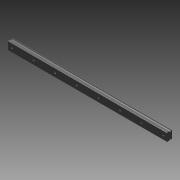
# Autodesk Inventor part: LU15AL294K2720100_rail
Saved by Autodesk Inventor 2011 SP1 (Build 150282100, 282)
## iProperties
Created: 2015-07-20
Part Number: LU15AL294K2720100_rail
Catalog Web Link: www.cadenas.de
Description: lu_rail-lu_rail
Vendor: NSK_RB
Document SubType Name: Modeling
Designer: PARTuser1
Manufacturer: NSK_RB
Mass: 37.8493 g
Surface Area: 162.952 cm^2
Volume: 37.8493 cm^3
Density: 1 g/cm^3
Category: PARTsolutions
Company: NSK_RB
Title: LU15AL
Author: Cadenas PARTsolutions
Comments: lu_rail
PSOL_IDENT_0: {$CADENAS_DATA\23d-libs\nsk_rb\nsk_linear_products\nsk_linear_guides\standard_series\lu_series\lu_al
PSOL_IDENT_1: _series\parts\lu_rail.prj},194 {VTYP=3D},{NB=LU15AL294K2720100_rail},{LINA=LU15AL},{NN=lu_rail},{DAT
PSOL_IDENT_2: E=17.04.2014 07:53:46},{GEOMDATE=17.04.2014 07:53:00},{VERSION=},{LINEID=740},{LINESUBID=-1},{WBVAR=
PSOL_IDENT_3: MAT,NOS,L0,G,POS1,POS2}  {NB=LU15AL294K2720100_rail},{LINA=LU15AL},{KT=DUMMY},{PN=LU15AL294K2720100_
PSOL_IDENT_4: rail},{MN=LU15AL},{ALG=LU15AL},{MNA=AL},{S=15},{MAT=K},{NOS=2},{L0=294},{G=7},{POS1=20},{POS2=100},{
PSOL_IDENT_5: MAT1='C','Special High carbon steel', 'K','Stainless steel'},{H=16.0},{E=4.0},{W2=8.5},{W=32},{L=43.
PSOL_IDENT_6: 600},{B=25},{J=20},{M=3.0},{TL=4.0},{B1=3.5},{L1=27.000},{J1=3.40},{K=12.0},{W1=15},{H1=9.5},{F=40},
PSOL_IDENT_7: {D=3.500},{DD=6.000},{HH=4.500},{B3=7.5},{G1=15.0},{GALGMIN=4},{GALGMAX=26.666667},{LMAX=1000},{LMIN=
PSOL_IDENT_8: 107.2},{NOMH=7},{POS1MIN=0},{POS1MAX=206.8},{POS2MIN=63.6},{POS2MAX=250.4},{DT=3.5},{DDT=6},{HHT=4.5
PSOL_IDENT_9: }
SUPPLIER: NSK_RB
ARTICLENO: LU15AL294K2720100_rail
BOMINFO: LU15AL
CREATOR: CADENAS GmbH
Autodesk Inventor part; units mm, degrees
sketch "Sketch_11" plane through (0, 0, 0) normal (1, 0, 0) x (0, 1, 0)
  line L0 (5, 7.5) -> (4.1225, 7.5)
  arc A0 (0.9321, 7.25) -> (4.1225, 7.5) centre (2.5175, 7.5) ccw
  line L1 (0.9321, 7.25) -> (0.25, 7.25)
  line L2 (0.25, 7.25) -> (0, 7.5)
  line L3 (0, 7.5) -> (-3.5, 7.5)
  line L4 (-3.5, 7.5) -> (-4, 7)
  line L5 (-4, 7) -> (-4, -6.9999)
  line L6 (-4, -6.9999) -> (-3.5, -7.5)
  line L7 (-3.5, -7.5) -> (0, -7.5)
  line L8 (0, -7.5) -> (0.25, -7.25)
  line L9 (0.25, -7.25) -> (0.9321, -7.25)
  arc A1 (4.1225, -7.5) -> (0.9321, -7.25) centre (2.5175, -7.5) ccw
  line L10 (4.1225, -7.5) -> (5, -7.5)
  line L11 (5, -7.5) -> (5.5, -7)
  line L12 (5.5, -7) -> (5.5, 7)
  line L13 (5.5, 7) -> (5, 7.5)
  constraints: 28 end point, 4 point on circle, 2 centre point
extrude "Extrusion1" add sketch "Sketch_11" along normal blind 294
sketch "Sketch_17" plane through (0, 0, 0) normal (0, 0, 1) x (1, 0, 0)
  line L0 (7, -4.5) -> (7, 6)
  line L1 (7, 6) -> (10, 6)
  line L2 (10, 6) -> (10, 1)
  line L3 (10, 1) -> (8.75, 1)
  line L4 (8.75, 1) -> (8.75, -4.5)
  line L5 (8.75, -4.5) -> (7, -4.5)
  line L6 (7, -4.5) -> (7, 6)
  constraints: 14 end point
revolve "Revolution1" cut sketch "Sketch_17" angle 360 about axis through (7, -4.5, 0) along (0, -1, 0)
pattern_linear "Rectangular Pattern1" count 8 spacing 40 along (1, 0, 0) of "Revolution1"
ref_plane "dummy_XY" through (7, -4, 0) normal (1, 0, 0) x (0, 0, -1)
ref_plane "dummy_YZ" through (7, -4, 0) normal (0, 0, -1) x (0, 1, 0)
ref_plane "dummy_ZX" through (7, -4, 0) normal (0, 1, 0) x (1, 0, 0)
ref_plane "slider_XY" through (20, 0, 0) normal (-1, 0, 0) x (0, 0, -1)
ref_plane "slider_YZ" through (20, 0, 0) normal (0, 0, -1) x (0, -1, 0)
ref_plane "slider_ZX" through (20, 0, 0) normal (0, -1, 0) x (-1, 0, 0)
ref_plane "slider2_XY" through (100, 0, 0) normal (-1, 0, 0) x (0, 0, -1)
ref_plane "slider2_YZ" through (100, 0, 0) normal (0, 0, -1) x (0, -1, 0)
ref_plane "slider2_ZX" through (100, 0, 0) normal (0, -1, 0) x (-1, 0, 0)
body "Solid1"
